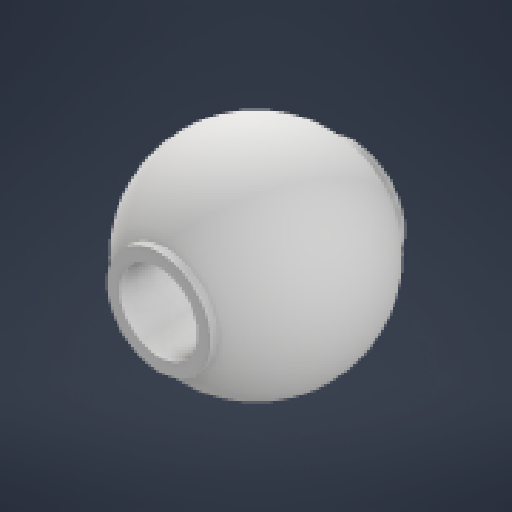
# Autodesk Inventor part: bALL
Saved by Autodesk Inventor 2024.3 (Build 283343000, 343)
## iProperties
Created: 2024-11-29
Part Number: bALL
Material: Generic
Document SubType Name: Modeling
Designer: MFil
Density: 1 g/cm^3
Appearance: Default
Author: MFil
Autodesk Inventor part; units mm, degrees
ref_plane "YZ Plane" through (0, 0, 0) normal (1, 0, 0) x (0, 1, 0)
ref_plane "XZ Plane" through (0, 0, 0) normal (0, 1, 0) x (-1, 0, 0)
ref_plane "XY Plane" through (0, 0, 0) normal (0, 0, 1) x (1, 0, 0)
sketch "Sketch1" plane through (0, 0, 0) normal (0, 0, 1) x (1, 0, 0)
  circle A0 centre (11, 6) radius 2
  circle A1 centre (11, 6) radius 1.5
  circle A2 centre (11, 6) radius 4
  line L0 (11, 10) -> (11, 1)
  point P0 (0, 0)
  point P1 (11, 2)
  dimension "d2" = 8
  dimension "d0" = 4
  dimension "d1" = 3
  constraints: 2 centre point, 2 coincident, 2 end point, 3 other
  measures "d0" diameter of A0
  measures "d1" diameter of A1
revolve "Revolution1" add sketch "Sketch1" angle 360 about axis through (11, 10, 0) along (0, -1, 0) picked at (12.8166, 5.8517) picked at (14.2832, 5.555) picked at (11.4875, 6.1113) contours A0 L0 A1 | A0 L0 A2 | A1 L0
extrude "Extrusion1" cut sketch "Sketch1" along normal mid plane 10 contours L0 A1 | A1 L0
extrude "Extrusion2" add sketch "Sketch1" along normal mid plane 7.5 contours A0 L0 A1 | L0 A1 A0
body "Solid1"
